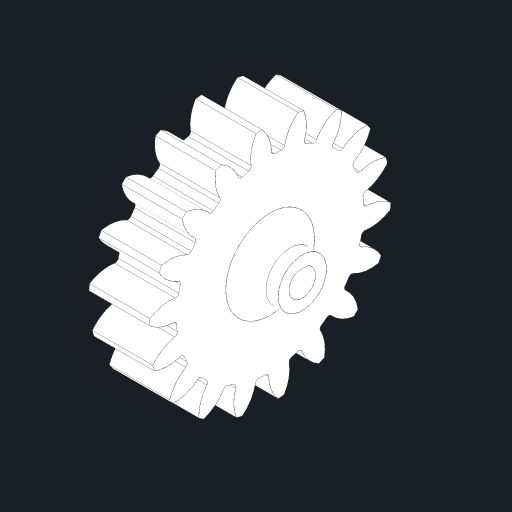
# Autodesk Inventor part: PINON DE TAPA PRINCIPAL
Saved by Autodesk Inventor 2024.3 (Build 283343000, 343)
## iProperties
Created: 2024-06-13
Part Number: PINON DE TAPA PRINCIPAL
Material: Generic
Document SubType Name: Modeling
Designer: Jhuliams
Density: 1 g/cm^3
Appearance: Default
Author: Jhuliams
Autodesk Inventor part; units mm, degrees
ref_plane "YZ Plane" through (0, 0, 0) normal (1, 0, 0) x (0, 1, 0)
ref_plane "XZ Plane" through (0, 0, 0) normal (0, 1, 0) x (-1, 0, 0)
ref_plane "XY Plane" through (0, 0, 0) normal (0, 0, 1) x (1, 0, 0)
sketch "Sketch1" plane through (0, 0, 0) normal (1, 0, 0) x (0, 1, 0)
  arc A0 (-3.216, -29.8271) -> (-1.751, -29.9489) centre (0, 0) ccw
  circle A1 centre (0, 0) radius 23.25
  line L0 (0, 0) -> (27, 0) construction
  arc A2 (-1.751, -29.9489) -> (0.5375, -23.2438) centre (-8.6776, -23.8416) ccw
  line L1 (0, 0) -> (27, 0) construction
  arc A3 (-4.3665, -22.8363) -> (-3.216, -29.8271) centre (4.6236, -24.9468) ccw
  arc A4 (3.7073, -22.9525) -> (7.1794, -29.1283) centre (12.8771, -21.861) ccw
  arc A5 (8.5977, -28.7416) -> (8.455, -21.6582) centre (0, -25.3717) ccw
  arc A6 (7.1794, -29.1283) -> (8.5977, -28.7416) centre (0, 0) ccw
  arc A7 (11.334, -20.3003) -> (16.7089, -24.9161) centre (19.5774, -16.1384) ccw
  arc A8 (17.9094, -24.0677) -> (15.3526, -17.4602) centre (8.6776, -23.8416) ccw
  arc A9 (16.7089, -24.9161) -> (17.9094, -24.0677) centre (0, 0) ccw
  arc A10 (17.5936, -15.1996) -> (24.223, -17.6987) centre (23.9164, -8.4692) ccw
  arc A11 (25.061, -16.4908) -> (20.3985, -11.1564) centre (16.3086, -19.4359) ccw
  arc A12 (24.223, -17.6987) -> (25.061, -16.4908) centre (0, 0) ccw
  arc A13 (21.7311, -8.2656) -> (28.8155, -8.3466) centre (25.3707, 0.2214) ccw
  arc A14 (29.1898, -6.925) -> (22.984, -3.5069) centre (21.9725, -12.6859) ccw
  arc A15 (28.8155, -8.3466) -> (29.1898, -6.925) centre (0, 0) ccw
  arc A16 (23.2476, -0.3347) -> (29.9324, 2.0123) centre (23.765, 8.8854) ccw
  arc A17 (29.7979, 3.4762) -> (22.7973, 4.5656) centre (24.9862, -4.4057) ccw
  arc A18 (29.9324, 2.0123) -> (29.7979, 3.4762) centre (0, 0) ccw
  arc A19 (21.9601, 7.6366) -> (27.439, 12.1284) centre (19.2928, 16.4776) ccw
  arc A20 (26.812, 13.458) -> (19.8609, 12.0874) centre (24.9862, 4.4057) ccw
  arc A21 (27.439, 12.1284) -> (26.812, 13.458) centre (0, 0) ccw
  arc A22 (18.0238, 14.6869) -> (21.6361, 20.7817) centre (12.4936, 22.0824) ccw
  arc A23 (20.5921, 21.8166) -> (14.529, 18.1513) centre (21.9725, 12.6859) ccw
  arc A24 (21.6361, 20.7817) -> (20.5921, 21.8166) centre (0, 0) ccw
  arc A25 (11.9136, 19.9657) -> (13.2235, 26.9284) centre (4.1875, 25.0237) ccw
  arc A26 (11.8885, 27.5438) -> (7.4447, 22.0259) centre (16.3086, 19.4359) ccw
  arc A27 (13.2235, 26.9284) -> (11.8885, 27.5438) centre (0, 0) ccw
  arc A28 (4.3665, 22.8363) -> (3.216, 29.8271) centre (-4.6236, 24.9468) ccw
  arc A29 (1.751, 29.9489) -> (-0.5375, 23.2438) centre (8.6776, 23.8416) ccw
  arc A30 (3.216, 29.8271) -> (1.751, 29.9489) centre (0, 0) ccw
  arc A31 (-3.7073, 22.9525) -> (-7.1794, 29.1283) centre (-12.8771, 21.861) ccw
  arc A32 (-8.5977, 28.7416) -> (-8.455, 21.6582) centre (0, 25.3717) ccw
  arc A33 (-7.1794, 29.1283) -> (-8.5977, 28.7416) centre (0, 0) ccw
  arc A34 (-11.334, 20.3003) -> (-16.7089, 24.9161) centre (-19.5774, 16.1384) ccw
  arc A35 (-17.9094, 24.0677) -> (-15.3526, 17.4602) centre (-8.6776, 23.8416) ccw
  arc A36 (-16.7089, 24.9161) -> (-17.9094, 24.0677) centre (0, 0) ccw
  arc A37 (-17.5936, 15.1996) -> (-24.223, 17.6987) centre (-23.9164, 8.4692) ccw
  arc A38 (-25.061, 16.4908) -> (-20.3985, 11.1564) centre (-16.3086, 19.4359) ccw
  arc A39 (-24.223, 17.6987) -> (-25.061, 16.4908) centre (0, 0) ccw
  arc A40 (-21.7311, 8.2656) -> (-28.8155, 8.3466) centre (-25.3707, -0.2214) ccw
  arc A41 (-29.1898, 6.925) -> (-22.984, 3.5069) centre (-21.9725, 12.6859) ccw
  arc A42 (-28.8155, 8.3466) -> (-29.1898, 6.925) centre (0, 0) ccw
  arc A43 (-23.2476, 0.3347) -> (-29.9324, -2.0123) centre (-23.765, -8.8854) ccw
  arc A44 (-29.7979, -3.4762) -> (-22.7973, -4.5656) centre (-24.9862, 4.4057) ccw
  arc A45 (-29.9324, -2.0123) -> (-29.7979, -3.4762) centre (0, 0) ccw
  arc A46 (-21.9601, -7.6366) -> (-27.439, -12.1284) centre (-19.2928, -16.4776) ccw
  arc A47 (-26.812, -13.458) -> (-19.8609, -12.0874) centre (-24.9862, -4.4057) ccw
  arc A48 (-27.439, -12.1284) -> (-26.812, -13.458) centre (0, 0) ccw
  arc A49 (-18.0238, -14.6869) -> (-21.6361, -20.7817) centre (-12.4936, -22.0824) ccw
  arc A50 (-20.5921, -21.8166) -> (-14.529, -18.1513) centre (-21.9725, -12.6859) ccw
  arc A51 (-21.6361, -20.7817) -> (-20.5921, -21.8166) centre (0, 0) ccw
  arc A52 (-11.9136, -19.9657) -> (-13.2235, -26.9284) centre (-4.1875, -25.0237) ccw
  arc A53 (-11.8885, -27.5438) -> (-7.4447, -22.0259) centre (-16.3086, -19.4359) ccw
  arc A54 (-13.2235, -26.9284) -> (-11.8885, -27.5438) centre (0, 0) ccw
  point P0 (14.529, 18.1513)
  point P1 (7.4447, 22.0259)
  point P2 (4.3665, 22.8363)
  point P3 (-0.5375, 23.2438)
  point P4 (-3.7073, 22.9525)
  point P5 (-11.334, 20.3003)
  point P6 (-15.3526, 17.4602)
  point P7 (-17.5936, 15.1996)
  point P8 (-22.984, 3.5069)
  point P9 (-23.2476, 0.3347)
  point P10 (-22.7973, -4.5656)
  point P11 (-21.9601, -7.6366)
  point P12 (-18.0238, -14.6869)
  point P13 (-14.529, -18.1513)
  point P14 (-7.4447, -22.0259)
  point P15 (-4.3665, -22.8363)
  point P16 (3.7073, -22.9525)
  point P17 (8.455, -21.6582)
  point P18 (11.334, -20.3003)
  point P19 (15.3526, -17.4602)
  point P20 (23.2476, -0.3347)
  point P21 (21.9601, 7.6366)
  point P22 (19.8609, 12.0874)
  dimension "d2" = 46.5
  dimension "d1" = 60
  dimension "d8" = 360
  constraints: 108 point on circle, 54 centre point, 4 end point, 2 horizontal, 1 coincident, 184 other
  measures "d1" diameter of A0
extrude "Extrusion1" add sketch "Sketch1" along normal blind 15
sketch "Sketch2" plane through (15, 0, 0) normal (1, 0, 0) x (0, 0, -1)
  circle A0 centre (0, 0) radius 2.6
  point P0 (-1.4107, 2.184)
  point P1 (1.4107, 2.184)
  point P2 (0, -2.6)
  dimension "d12" = 5.2
  constraints: 3 point on circle, 1 centre point, 1 coincident, 1 vertical alignment
  measures "d12" diameter of A0
extrude "Extrusion2" cut sketch "Sketch2" against normal blind 15
fillet "Fillet1" radius 0.78 2 edges at (7.5, 19.8609, 12.0874) (7.5, 18.0238, 14.6869)
pattern_circular "Circular Pattern1" count 18 over 360 about axis through (15, 0, 0) along (-1, 0, 0) of "Fillet1"
sketch "Sketch3" plane through (15, 0, 0) normal (1, 0, 0) x (0, 0, -1)
  circle A0 centre (0, 0) radius 2.6 projected
  arc A1 (-21.8166, 20.5921) -> (-18.7279, 14.9889) centre (-12.6859, 21.9725) ccw projected
  arc A2 (-18.6137, 13.9317) -> (-18.7279, 14.9889) centre (-19.2382, 14.399) ccw projected
  arc A3 (-18.6137, 13.9317) -> (-19.5681, 12.556) centre (0, 0) ccw projected
  arc A4 (-20.5983, 12.2926) -> (-19.5681, 12.556) centre (-20.2245, 12.9772) ccw projected
  arc A5 (-20.5983, 12.2926) -> (-26.9284, 13.2235) centre (-25.0237, 4.1875) ccw projected
  arc A6 (-26.9284, 13.2235) -> (-27.5438, 11.8885) centre (0, 0) ccw projected
  arc A7 (-27.5438, 11.8885) -> (-22.7249, 7.6797) centre (-19.4359, 16.3086) ccw projected
  arc A8 (-22.2561, 6.7252) -> (-22.7249, 7.6797) centre (-23.0028, 6.9508) ccw projected
  arc A9 (-22.2561, 6.7252) -> (-22.6824, 5.1061) centre (0, 0) ccw projected
  arc A10 (-23.5604, 4.5063) -> (-22.6824, 5.1061) centre (-23.4433, 5.2774) ccw projected
  arc A11 (-23.5604, 4.5063) -> (-29.8271, 3.216) centre (-24.9468, -4.6236) ccw projected
  arc A12 (-29.8271, 3.216) -> (-29.9489, 1.751) centre (0, 0) ccw projected
  arc A13 (-29.9489, 1.751) -> (-23.9811, -0.5559) centre (-23.8416, 8.6776) ccw projected
  arc A14 (-23.2141, -1.2924) -> (-23.9811, -0.5559) centre (-23.9928, -1.3358) ccw projected
  arc A15 (-23.2141, -1.2924) -> (-23.0609, -2.9597) centre (0, 0) ccw projected
  arc A16 (-23.6808, -3.8237) -> (-23.0609, -2.9597) centre (-23.8345, -3.0589) ccw projected
  arc A17 (-23.6808, -3.8237) -> (-29.1283, -7.1794) centre (-21.861, -12.8771) ccw projected
  arc A18 (-29.1283, -7.1794) -> (-28.7416, -8.5977) centre (0, 0) ccw projected
  arc A19 (-28.7416, -8.5977) -> (-22.3447, -8.7243) centre (-25.3717, 0) ccw projected
  arc A20 (-21.372, -9.1541) -> (-22.3447, -8.7243) centre (-22.089, -9.4612) ccw projected
  arc A21 (-21.372, -9.1541) -> (-20.6579, -10.6684) centre (0, 0) ccw projected
  arc A22 (-20.9449, -11.6924) -> (-20.6579, -10.6684) centre (-21.3509, -11.0264) ccw projected
  arc A23 (-20.9449, -11.6924) -> (-24.9161, -16.7089) centre (-16.1384, -19.5774) ccw projected
  arc A24 (-24.9161, -16.7089) -> (-24.0677, -17.9094) centre (0, 0) ccw projected
  arc A25 (-24.0677, -17.9094) -> (-18.0133, -15.8405) centre (-23.8416, -8.6776) ccw projected
  arc A26 (-16.9522, -15.9117) -> (-18.0133, -15.8405) centre (-17.521, -16.4456) ccw projected
  arc A27 (-16.9522, -15.9117) -> (-15.7632, -17.0905) centre (0, 0) ccw projected
  arc A28 (-15.6827, -18.1508) -> (-15.7632, -17.0905) centre (-16.292, -17.6638) ccw projected
  arc A29 (-15.6827, -18.1508) -> (-17.6987, -24.223) centre (-8.4692, -23.9164) ccw projected
  arc A30 (-17.6987, -24.223) -> (-16.4908, -25.061) centre (0, 0) ccw projected
  arc A31 (-16.4908, -25.061) -> (-11.5091, -21.0461) centre (-19.4359, -16.3086) ccw projected
  arc A32 (-10.4878, -20.7502) -> (-11.5091, -21.0461) centre (-10.8396, -21.4463) ccw projected
  arc A33 (-10.4878, -20.7502) -> (-8.9673, -21.4511) centre (0, 0) ccw projected
  arc A34 (-8.529, -22.42) -> (-8.9673, -21.4511) centre (-9.2681, -22.1708) ccw projected
  arc A35 (-8.529, -22.42) -> (-8.3466, -28.8155) centre (0.2214, -25.3707) ccw projected
  arc A36 (-8.3466, -28.8155) -> (-6.925, -29.1898) centre (0, 0) ccw projected
  arc A37 (-6.925, -29.1898) -> (-3.6169, -23.7133) centre (-12.6859, -21.9725) ccw projected
  arc A38 (-2.7583, -23.0858) -> (-3.6169, -23.7133) centre (-2.8508, -23.8603) ccw projected
  arc A39 (-2.7583, -23.0858) -> (-1.0898, -23.2244) centre (0, 0) ccw projected
  arc A40 (-0.3466, -23.985) -> (-1.0898, -23.2244) centre (-1.1263, -24.0036) ccw projected
  arc A41 (-0.3466, -23.985) -> (2.0123, -29.9324) centre (8.8854, -23.765) ccw projected
  arc A42 (2.0123, -29.9324) -> (3.4762, -29.7979) centre (0, 0) ccw projected
  arc A43 (3.4762, -29.7979) -> (4.7117, -23.5202) centre (-4.4057, -24.9862) ccw projected
  arc A44 (5.3039, -22.637) -> (4.7117, -23.5202) centre (5.4818, -23.3964) ccw projected
  arc A45 (5.3039, -22.637) -> (6.9192, -22.1966) centre (0, 0) ccw projected
  arc A46 (7.8777, -22.6571) -> (6.9192, -22.1966) centre (7.1513, -22.9412) ccw projected
  arc A47 (7.8777, -22.6571) -> (12.1284, -27.439) centre (16.4776, -19.2928) ccw projected
  arc A48 (12.1284, -27.439) -> (13.458, -26.812) centre (0, 0) ccw projected
  arc A49 (13.458, -26.812) -> (12.4719, -20.4903) centre (4.4057, -24.9862) ccw projected
  arc A50 (12.7263, -19.4578) -> (12.4719, -20.4903) centre (13.1532, -20.1105) ccw projected
  arc A51 (12.7263, -19.4578) -> (14.0936, -18.4915) centre (0, 0) ccw projected
  arc A52 (15.1518, -18.5963) -> (14.0936, -18.4915) centre (14.5664, -19.1118) ccw projected
  arc A53 (15.1518, -18.5963) -> (20.7817, -21.6361) centre (22.0824, -12.4936) ccw projected
  arc A54 (20.7817, -21.6361) -> (21.8166, -20.5921) centre (0, 0) ccw projected
  arc A55 (21.8166, -20.5921) -> (18.7279, -14.9889) centre (12.6859, -21.9725) ccw projected
  arc A56 (18.6137, -13.9317) -> (18.7279, -14.9889) centre (19.2382, -14.399) ccw projected
  arc A57 (18.6137, -13.9317) -> (19.5681, -12.556) centre (0, 0) ccw projected
  arc A58 (20.5983, -12.2926) -> (19.5681, -12.556) centre (20.2245, -12.9772) ccw projected
  arc A59 (20.5983, -12.2926) -> (26.9284, -13.2235) centre (25.0237, -4.1875) ccw projected
  arc A60 (26.9284, -13.2235) -> (27.5438, -11.8885) centre (0, 0) ccw projected
  arc A61 (27.5438, -11.8885) -> (22.7249, -7.6797) centre (19.4359, -16.3086) ccw projected
  arc A62 (22.2561, -6.7252) -> (22.7249, -7.6797) centre (23.0028, -6.9508) ccw projected
  arc A63 (22.2561, -6.7252) -> (22.6824, -5.1061) centre (0, 0) ccw projected
  arc A64 (23.5604, -4.5063) -> (22.6824, -5.1061) centre (23.4433, -5.2774) ccw projected
  arc A65 (23.5604, -4.5063) -> (29.8271, -3.216) centre (24.9468, 4.6236) ccw projected
  arc A66 (29.8271, -3.216) -> (29.9489, -1.751) centre (0, 0) ccw projected
  arc A67 (29.9489, -1.751) -> (23.9811, 0.5559) centre (23.8416, -8.6776) ccw projected
  arc A68 (23.2141, 1.2924) -> (23.9811, 0.5559) centre (23.9928, 1.3358) ccw projected
  arc A69 (23.2141, 1.2924) -> (23.0609, 2.9597) centre (0, 0) ccw projected
  arc A70 (23.6808, 3.8237) -> (23.0609, 2.9597) centre (23.8345, 3.0589) ccw projected
  arc A71 (23.6808, 3.8237) -> (29.1283, 7.1794) centre (21.861, 12.8771) ccw projected
  arc A72 (29.1283, 7.1794) -> (28.7416, 8.5977) centre (0, 0) ccw projected
  arc A73 (28.7416, 8.5977) -> (22.3447, 8.7243) centre (25.3717, 0) ccw projected
  arc A74 (21.372, 9.1541) -> (22.3447, 8.7243) centre (22.089, 9.4612) ccw projected
  arc A75 (21.372, 9.1541) -> (20.6579, 10.6684) centre (0, 0) ccw projected
  arc A76 (20.9449, 11.6924) -> (20.6579, 10.6684) centre (21.3509, 11.0264) ccw projected
  arc A77 (20.9449, 11.6924) -> (24.9161, 16.7089) centre (16.1384, 19.5774) ccw projected
  arc A78 (24.9161, 16.7089) -> (24.0677, 17.9094) centre (0, 0) ccw projected
  arc A79 (24.0677, 17.9094) -> (18.0133, 15.8405) centre (23.8416, 8.6776) ccw projected
  arc A80 (16.9522, 15.9117) -> (18.0133, 15.8405) centre (17.521, 16.4456) ccw projected
  arc A81 (16.9522, 15.9117) -> (15.7632, 17.0905) centre (0, 0) ccw projected
  arc A82 (15.6827, 18.1508) -> (15.7632, 17.0905) centre (16.292, 17.6638) ccw projected
  arc A83 (15.6827, 18.1508) -> (17.6987, 24.223) centre (8.4692, 23.9164) ccw projected
  arc A84 (17.6987, 24.223) -> (16.4908, 25.061) centre (0, 0) ccw projected
  arc A85 (16.4908, 25.061) -> (11.5091, 21.0461) centre (19.4359, 16.3086) ccw projected
  arc A86 (10.4878, 20.7502) -> (11.5091, 21.0461) centre (10.8396, 21.4463) ccw projected
  arc A87 (10.4878, 20.7502) -> (8.9673, 21.4511) centre (0, 0) ccw projected
  arc A88 (8.529, 22.42) -> (8.9673, 21.4511) centre (9.2681, 22.1708) ccw projected
  arc A89 (8.529, 22.42) -> (8.3466, 28.8155) centre (-0.2214, 25.3707) ccw projected
  arc A90 (8.3466, 28.8155) -> (6.925, 29.1898) centre (0, 0) ccw projected
  arc A91 (6.925, 29.1898) -> (3.6169, 23.7133) centre (12.6859, 21.9725) ccw projected
  arc A92 (2.7583, 23.0858) -> (3.6169, 23.7133) centre (2.8508, 23.8603) ccw projected
  arc A93 (2.7583, 23.0858) -> (1.0898, 23.2244) centre (0, 0) ccw projected
  arc A94 (0.3466, 23.985) -> (1.0898, 23.2244) centre (1.1263, 24.0036) ccw projected
  arc A95 (0.3466, 23.985) -> (-2.0123, 29.9324) centre (-8.8854, 23.765) ccw projected
  arc A96 (-2.0123, 29.9324) -> (-3.4762, 29.7979) centre (0, 0) ccw projected
  arc A97 (-3.4762, 29.7979) -> (-4.7117, 23.5202) centre (4.4057, 24.9862) ccw projected
  arc A98 (-5.3039, 22.637) -> (-4.7117, 23.5202) centre (-5.4818, 23.3964) ccw projected
  arc A99 (-5.3039, 22.637) -> (-6.9192, 22.1966) centre (0, 0) ccw projected
  arc A100 (-7.8777, 22.6571) -> (-6.9192, 22.1966) centre (-7.1513, 22.9412) ccw projected
  arc A101 (-7.8777, 22.6571) -> (-12.1284, 27.439) centre (-16.4776, 19.2928) ccw projected
  arc A102 (-12.1284, 27.439) -> (-13.458, 26.812) centre (0, 0) ccw projected
  arc A103 (-13.458, 26.812) -> (-12.4719, 20.4903) centre (-4.4057, 24.9862) ccw projected
  arc A104 (-12.7263, 19.4578) -> (-12.4719, 20.4903) centre (-13.1532, 20.1105) ccw projected
  arc A105 (-12.7263, 19.4578) -> (-14.0936, 18.4915) centre (0, 0) ccw projected
  arc A106 (-15.1518, 18.5963) -> (-14.0936, 18.4915) centre (-14.5664, 19.1118) ccw projected
  arc A107 (-15.1518, 18.5963) -> (-20.7817, 21.6361) centre (-22.0824, 12.4936) ccw projected
  arc A108 (-20.7817, 21.6361) -> (-21.8166, 20.5921) centre (0, 0) ccw projected
  circle A109 centre (0, 0) radius 6
  dimension "d22" = 12
  constraints: 1 centre point, 1 coincident
  measures "d22" diameter of A109
extrude "Extrusion3" add sketch "Sketch3" along normal blind 8 contours A109
fillet "Fillet2" radius 5 1 edges at (15, 0, 6)
sketch "Sketch4" plane through (0, 0, 0) normal (-1, 0, 0) x (0, 0, 1)
  circle A0 centre (0, 0) radius 2.6 projected
  arc A1 (18.7279, 14.9889) -> (21.8166, 20.5921) centre (12.6859, 21.9725) ccw projected
  arc A2 (21.8166, 20.5921) -> (20.7817, 21.6361) centre (0, 0) ccw projected
  arc A3 (20.7817, 21.6361) -> (15.1518, 18.5963) centre (22.0824, 12.4936) ccw projected
  arc A4 (14.0936, 18.4915) -> (15.1518, 18.5963) centre (14.5664, 19.1118) ccw projected
  arc A5 (14.0936, 18.4915) -> (12.7263, 19.4578) centre (0, 0) ccw projected
  arc A6 (12.4719, 20.4903) -> (12.7263, 19.4578) centre (13.1532, 20.1105) ccw projected
  arc A7 (12.4719, 20.4903) -> (13.458, 26.812) centre (4.4057, 24.9862) ccw projected
  arc A8 (13.458, 26.812) -> (12.1284, 27.439) centre (0, 0) ccw projected
  arc A9 (12.1284, 27.439) -> (7.8777, 22.6571) centre (16.4776, 19.2928) ccw projected
  arc A10 (6.9192, 22.1966) -> (7.8777, 22.6571) centre (7.1513, 22.9412) ccw projected
  arc A11 (6.9192, 22.1966) -> (5.3039, 22.637) centre (0, 0) ccw projected
  arc A12 (4.7117, 23.5202) -> (5.3039, 22.637) centre (5.4818, 23.3964) ccw projected
  arc A13 (4.7117, 23.5202) -> (3.4762, 29.7979) centre (-4.4057, 24.9862) ccw projected
  arc A14 (3.4762, 29.7979) -> (2.0123, 29.9324) centre (0, 0) ccw projected
  arc A15 (2.0123, 29.9324) -> (-0.3466, 23.985) centre (8.8854, 23.765) ccw projected
  arc A16 (-1.0898, 23.2244) -> (-0.3466, 23.985) centre (-1.1263, 24.0036) ccw projected
  arc A17 (-1.0898, 23.2244) -> (-2.7583, 23.0858) centre (0, 0) ccw projected
  arc A18 (-3.6169, 23.7133) -> (-2.7583, 23.0858) centre (-2.8508, 23.8603) ccw projected
  arc A19 (-3.6169, 23.7133) -> (-6.925, 29.1898) centre (-12.6859, 21.9725) ccw projected
  arc A20 (-6.925, 29.1898) -> (-8.3466, 28.8155) centre (0, 0) ccw projected
  arc A21 (-8.3466, 28.8155) -> (-8.529, 22.42) centre (0.2214, 25.3707) ccw projected
  arc A22 (-8.9673, 21.4511) -> (-8.529, 22.42) centre (-9.2681, 22.1708) ccw projected
  arc A23 (-8.9673, 21.4511) -> (-10.4878, 20.7502) centre (0, 0) ccw projected
  arc A24 (-11.5091, 21.0461) -> (-10.4878, 20.7502) centre (-10.8396, 21.4463) ccw projected
  arc A25 (-11.5091, 21.0461) -> (-16.4908, 25.061) centre (-19.4359, 16.3086) ccw projected
  arc A26 (-16.4908, 25.061) -> (-17.6987, 24.223) centre (0, 0) ccw projected
  arc A27 (-17.6987, 24.223) -> (-15.6827, 18.1508) centre (-8.4692, 23.9164) ccw projected
  arc A28 (-15.7632, 17.0905) -> (-15.6827, 18.1508) centre (-16.292, 17.6638) ccw projected
  arc A29 (-15.7632, 17.0905) -> (-16.9522, 15.9117) centre (0, 0) ccw projected
  arc A30 (-18.0133, 15.8405) -> (-16.9522, 15.9117) centre (-17.521, 16.4456) ccw projected
  arc A31 (-18.0133, 15.8405) -> (-24.0677, 17.9094) centre (-23.8416, 8.6776) ccw projected
  arc A32 (-24.0677, 17.9094) -> (-24.9161, 16.7089) centre (0, 0) ccw projected
  arc A33 (-24.9161, 16.7089) -> (-20.9449, 11.6924) centre (-16.1384, 19.5774) ccw projected
  arc A34 (-20.6579, 10.6684) -> (-20.9449, 11.6924) centre (-21.3509, 11.0264) ccw projected
  arc A35 (-20.6579, 10.6684) -> (-21.372, 9.1541) centre (0, 0) ccw projected
  arc A36 (-22.3447, 8.7243) -> (-21.372, 9.1541) centre (-22.089, 9.4612) ccw projected
  arc A37 (-22.3447, 8.7243) -> (-28.7416, 8.5977) centre (-25.3717, 0) ccw projected
  arc A38 (-28.7416, 8.5977) -> (-29.1283, 7.1794) centre (0, 0) ccw projected
  arc A39 (-29.1283, 7.1794) -> (-23.6808, 3.8237) centre (-21.861, 12.8771) ccw projected
  arc A40 (-23.0609, 2.9597) -> (-23.6808, 3.8237) centre (-23.8345, 3.0589) ccw projected
  arc A41 (-23.0609, 2.9597) -> (-23.2141, 1.2924) centre (0, 0) ccw projected
  arc A42 (-23.9811, 0.5559) -> (-23.2141, 1.2924) centre (-23.9928, 1.3358) ccw projected
  arc A43 (-23.9811, 0.5559) -> (-29.9489, -1.751) centre (-23.8416, -8.6776) ccw projected
  arc A44 (-29.9489, -1.751) -> (-29.8271, -3.216) centre (0, 0) ccw projected
  arc A45 (-29.8271, -3.216) -> (-23.5604, -4.5063) centre (-24.9468, 4.6236) ccw projected
  arc A46 (-22.6824, -5.1061) -> (-23.5604, -4.5063) centre (-23.4433, -5.2774) ccw projected
  arc A47 (-22.6824, -5.1061) -> (-22.2561, -6.7252) centre (0, 0) ccw projected
  arc A48 (-22.7249, -7.6797) -> (-22.2561, -6.7252) centre (-23.0028, -6.9508) ccw projected
  arc A49 (-22.7249, -7.6797) -> (-27.5438, -11.8885) centre (-19.4359, -16.3086) ccw projected
  arc A50 (-27.5438, -11.8885) -> (-26.9284, -13.2235) centre (0, 0) ccw projected
  arc A51 (-26.9284, -13.2235) -> (-20.5983, -12.2926) centre (-25.0237, -4.1875) ccw projected
  arc A52 (-19.5681, -12.556) -> (-20.5983, -12.2926) centre (-20.2245, -12.9772) ccw projected
  arc A53 (-19.5681, -12.556) -> (-18.6137, -13.9317) centre (0, 0) ccw projected
  arc A54 (-18.7279, -14.9889) -> (-18.6137, -13.9317) centre (-19.2382, -14.399) ccw projected
  arc A55 (-18.7279, -14.9889) -> (-21.8166, -20.5921) centre (-12.6859, -21.9725) ccw projected
  arc A56 (-21.8166, -20.5921) -> (-20.7817, -21.6361) centre (0, 0) ccw projected
  arc A57 (-20.7817, -21.6361) -> (-15.1518, -18.5963) centre (-22.0824, -12.4936) ccw projected
  arc A58 (-14.0936, -18.4915) -> (-15.1518, -18.5963) centre (-14.5664, -19.1118) ccw projected
  arc A59 (-14.0936, -18.4915) -> (-12.7263, -19.4578) centre (0, 0) ccw projected
  arc A60 (-12.4719, -20.4903) -> (-12.7263, -19.4578) centre (-13.1532, -20.1105) ccw projected
  arc A61 (-12.4719, -20.4903) -> (-13.458, -26.812) centre (-4.4057, -24.9862) ccw projected
  arc A62 (-13.458, -26.812) -> (-12.1284, -27.439) centre (0, 0) ccw projected
  arc A63 (-12.1284, -27.439) -> (-7.8777, -22.6571) centre (-16.4776, -19.2928) ccw projected
  arc A64 (-6.9192, -22.1966) -> (-7.8777, -22.6571) centre (-7.1513, -22.9412) ccw projected
  arc A65 (-6.9192, -22.1966) -> (-5.3039, -22.637) centre (0, 0) ccw projected
  arc A66 (-4.7117, -23.5202) -> (-5.3039, -22.637) centre (-5.4818, -23.3964) ccw projected
  arc A67 (-4.7117, -23.5202) -> (-3.4762, -29.7979) centre (4.4057, -24.9862) ccw projected
  arc A68 (-3.4762, -29.7979) -> (-2.0123, -29.9324) centre (0, 0) ccw projected
  arc A69 (-2.0123, -29.9324) -> (0.3466, -23.985) centre (-8.8854, -23.765) ccw projected
  arc A70 (1.0898, -23.2244) -> (0.3466, -23.985) centre (1.1263, -24.0036) ccw projected
  arc A71 (1.0898, -23.2244) -> (2.7583, -23.0858) centre (0, 0) ccw projected
  arc A72 (3.6169, -23.7133) -> (2.7583, -23.0858) centre (2.8508, -23.8603) ccw projected
  arc A73 (3.6169, -23.7133) -> (6.925, -29.1898) centre (12.6859, -21.9725) ccw projected
  arc A74 (6.925, -29.1898) -> (8.3466, -28.8155) centre (0, 0) ccw projected
  arc A75 (8.3466, -28.8155) -> (8.529, -22.42) centre (-0.2214, -25.3707) ccw projected
  arc A76 (8.9673, -21.4511) -> (8.529, -22.42) centre (9.2681, -22.1708) ccw projected
  arc A77 (8.9673, -21.4511) -> (10.4878, -20.7502) centre (0, 0) ccw projected
  arc A78 (11.5091, -21.0461) -> (10.4878, -20.7502) centre (10.8396, -21.4463) ccw projected
  arc A79 (11.5091, -21.0461) -> (16.4908, -25.061) centre (19.4359, -16.3086) ccw projected
  arc A80 (16.4908, -25.061) -> (17.6987, -24.223) centre (0, 0) ccw projected
  arc A81 (17.6987, -24.223) -> (15.6827, -18.1508) centre (8.4692, -23.9164) ccw projected
  arc A82 (15.7632, -17.0905) -> (15.6827, -18.1508) centre (16.292, -17.6638) ccw projected
  arc A83 (15.7632, -17.0905) -> (16.9522, -15.9117) centre (0, 0) ccw projected
  arc A84 (18.0133, -15.8405) -> (16.9522, -15.9117) centre (17.521, -16.4456) ccw projected
  arc A85 (18.0133, -15.8405) -> (24.0677, -17.9094) centre (23.8416, -8.6776) ccw projected
  arc A86 (24.0677, -17.9094) -> (24.9161, -16.7089) centre (0, 0) ccw projected
  arc A87 (24.9161, -16.7089) -> (20.9449, -11.6924) centre (16.1384, -19.5774) ccw projected
  arc A88 (20.6579, -10.6684) -> (20.9449, -11.6924) centre (21.3509, -11.0264) ccw projected
  arc A89 (20.6579, -10.6684) -> (21.372, -9.1541) centre (0, 0) ccw projected
  arc A90 (22.3447, -8.7243) -> (21.372, -9.1541) centre (22.089, -9.4612) ccw projected
  arc A91 (22.3447, -8.7243) -> (28.7416, -8.5977) centre (25.3717, 0) ccw projected
  arc A92 (28.7416, -8.5977) -> (29.1283, -7.1794) centre (0, 0) ccw projected
  arc A93 (29.1283, -7.1794) -> (23.6808, -3.8237) centre (21.861, -12.8771) ccw projected
  arc A94 (23.0609, -2.9597) -> (23.6808, -3.8237) centre (23.8345, -3.0589) ccw projected
  arc A95 (23.0609, -2.9597) -> (23.2141, -1.2924) centre (0, 0) ccw projected
  arc A96 (23.9811, -0.5559) -> (23.2141, -1.2924) centre (23.9928, -1.3358) ccw projected
  arc A97 (23.9811, -0.5559) -> (29.9489, 1.751) centre (23.8416, 8.6776) ccw projected
  arc A98 (29.9489, 1.751) -> (29.8271, 3.216) centre (0, 0) ccw projected
  arc A99 (29.8271, 3.216) -> (23.5604, 4.5063) centre (24.9468, -4.6236) ccw projected
  arc A100 (22.6824, 5.1061) -> (23.5604, 4.5063) centre (23.4433, 5.2774) ccw projected
  arc A101 (22.6824, 5.1061) -> (22.2561, 6.7252) centre (0, 0) ccw projected
  arc A102 (22.7249, 7.6797) -> (22.2561, 6.7252) centre (23.0028, 6.9508) ccw projected
  arc A103 (22.7249, 7.6797) -> (27.5438, 11.8885) centre (19.4359, 16.3086) ccw projected
  arc A104 (27.5438, 11.8885) -> (26.9284, 13.2235) centre (0, 0) ccw projected
  arc A105 (26.9284, 13.2235) -> (20.5983, 12.2926) centre (25.0237, 4.1875) ccw projected
  arc A106 (19.5681, 12.556) -> (20.5983, 12.2926) centre (20.2245, 12.9772) ccw projected
  arc A107 (19.5681, 12.556) -> (18.6137, 13.9317) centre (0, 0) ccw projected
  arc A108 (18.7279, 14.9889) -> (18.6137, 13.9317) centre (19.2382, 14.399) ccw projected
  circle A109 centre (0, 0) radius 3.3
  line L0 (-1.39, 2.993) -> (1.39, 2.993)
  dimension "d26" = 6.6
  constraints: 2 end point, 2 point on circle, 1 centre point, 1 coincident, 1 horizontal
  measures "d26" diameter of A109
extrude "Extrusion4" cut sketch "Sketch4" against normal through all contours A109 L0 picked at (-0.1045, 2.8557)
body "Solid1"
